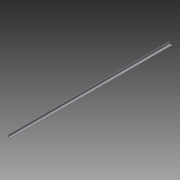
# Autodesk Inventor part: Y_Rail-SquareBar-Rev3
Saved by Autodesk Inventor 2015 (Build 190159000, 159)
## iProperties
Created: 2017-01-10
Part Number: Y_Rail-SquareBar-Rev3
Material: Generic
Document SubType Name: Modeling
Designer: Guy
Density: 1 g/cm^3
Appearance: Default
Mass: 222.064 g
Surface Area: 1563.73 cm^2
Volume: 222.064 cm^3
Author: Guy
Autodesk Inventor part; units mm, degrees
ref_plane "YZ Plane" through (0, 0, 0) normal (1, 0, 0) x (0, 1, 0)
ref_plane "XZ Plane" through (0, 0, 0) normal (0, 1, 0) x (-1, 0, 0)
ref_plane "XY Plane" through (0, 0, 0) normal (0, 0, 1) x (1, 0, 0)
sketch "Sketch1" plane through (0, 0, 0) normal (0, 0, 1) x (1, 0, 0)
  line L0 (0, 0) -> (0, 25.5)
  line L1 (0, 25.5) -> (3.2, 25.5)
  line L2 (3.2, 25.5) -> (3.2, 3.2)
  line L3 (3.2, 3.2) -> (25.5, 3.2)
  line L4 (25.5, 3.2) -> (25.5, 0)
  line L5 (25.5, 0) -> (0, 0)
  dimension "d0" = 25.5
  dimension "d1" = 25.5
  dimension "d2" = 3.2
  dimension "d3" = 3.2
  constraints: 12 end point, 5 perpendicular, 1 vertical
  measures "d0" distance between parallel lines of L0 L4
  measures "d1" distance between parallel lines of L5 L1
  measures "d2" distance between parallel lines of L0 L2
  measures "d3" distance between parallel lines of L5 L3
extrude "Extrusion1" add sketch "Sketch1" along normal blind 1712.786
sketch "Sketch3" plane through (3.2, 3.2, 0) normal (1, 0, 0) x (0, 0, -1)
  line L0 (0, 22.3) -> (0, 0) projected
  line L1 (0, 22.3) -> (-1712.786, 22.3) projected
  line L2 (-1712.786, 0) -> (-1712.786, 22.3) projected
  line L3 (0, 0) -> (-1712.786, 0) projected
  circle A0 centre (-11.925, 7.3) radius 2.425
  circle A1 centre (-30.325, 7.3) radius 2.425
  circle A2 centre (-1702.786, 7.3) radius 2.425
  circle A3 centre (-1684.386, 7.3) radius 2.425
  point P0 (0, -3.2)
  dimension "d20" = 4.85
  dimension "d21" = 4.85
  dimension "d22" = 15
  dimension "d24" = 11.925
  dimension "d28" = 4.85
  dimension "d30" = 10
  dimension "d32" = 15
  dimension "d33" = 18.4
  dimension "d34" = 18.4
  dimension "d35" = 15
  dimension "d36" = 15
  dimension "d37" = 4.85
  constraints: 4 centre point
  measures "d20" diameter of A1
  measures "d21" diameter of A0
  measures "d22" distance from line of L1 A0.centre
  measures "d24" distance from line of L0 A0.centre
  measures "d28" diameter of A2
  measures "d30" distance from line of L2 A2.centre
  measures "d32" distance from line of L1 A2.centre
  measures "d33" distance of A3.centre A2.centre
  measures "d34" distance of A1.centre A0.centre
  measures "d35" distance from line of A1.centre L1
  measures "d36" distance from line of A3.centre L1
  measures "d37" diameter of A3
extrude "Extrusion3" cut sketch "Sketch3" against normal blind 1300 contours A0 | A1 | A2 | A3
body "Solid1"
